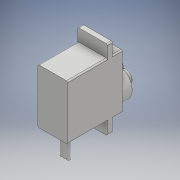
# Autodesk Inventor part: 9g-micro-server
Saved by Autodesk Inventor 2018 (Build 220112000, 112)
## iProperties
Created: 2017-10-10
Part Number: 9g-micro-server
Material: Generic
Document SubType Name: Modeling
Designer: leo2a
Density: 1 g/cm^3
Appearance: Default
Author: leo2a
Autodesk Inventor part; units mm, degrees
ref_plane "YZ Plane" through (0, 0, 0) normal (1, 0, 0) x (0, 1, 0)
ref_plane "XZ Plane" through (0, 0, 0) normal (0, 1, 0) x (-1, 0, 0)
ref_plane "XY Plane" through (0, 0, 0) normal (0, 0, 1) x (1, 0, 0)
sketch "Sketch1" plane through (0, 0, 0) normal (0, 1, 0) x (-1, 0, 0)
  line L0 (-6, 11) -> (-6, -11)
  line L1 (-6, -11) -> (6, -11)
  line L2 (6, -11) -> (6, 11)
  line L3 (6, 11) -> (-6, 11)
  line L4 (-6, 11) -> (6, -11) construction
  line L5 (-6, -11) -> (6, 11) construction
  point P0 (0, 0)
  dimension "d0" = 22
  dimension "d1" = 12
  constraints: 12 end point, 2 midpoint, 2 parallel, 1 perpendicular, 1 vertical
  measures "d0" distance of L0.start L0.end
  measures "d1" distance of L1.end L0.end
extrude "Extrusion1" add sketch "Sketch1" along normal blind 16
sketch "Sketch2" plane through (0, 16, 0) normal (0, 1, 0) x (1, 0, 0)
  line L0 (6, -16) -> (6, 16)
  line L1 (6, 16) -> (-6, 16)
  line L2 (-6, 16) -> (-6, -16)
  line L3 (-6, -16) -> (6, -16)
  line L4 (6, -16) -> (-6, 16) construction
  line L5 (6, 16) -> (-6, -16) construction
  point P0 (0, 0)
  dimension "d4" = 32
  constraints: 12 end point, 2 midpoint, 2 parallel, 1 perpendicular, 1 vertical
  measures "d4" distance of L0.start L0.end
extrude "Extrusion2" add sketch "Sketch2" along normal blind 2
sketch "Sketch3" plane through (0, 18, 0) normal (0, 1, 0) x (1, 0, 0)
  line L0 (6, -11) -> (6, 11)
  line L1 (6, 11) -> (-6, 11)
  line L2 (-6, 11) -> (-6, -11)
  line L3 (-6, -11) -> (6, -11)
  line L4 (6, -11) -> (-6, 11) construction
  line L5 (6, 11) -> (-6, -11) construction
  point P0 (0, 0)
  constraints: 12 end point, 2 midpoint, 2 parallel, 1 perpendicular
extrude "Extrusion3" add sketch "Sketch3" along normal blind 4
sketch "Sketch4" plane through (0, 22, 0) normal (0, 1, 0) x (1, 0, 0)
  line L0 (6, 11) -> (-6, 11) projected
  line L1 (0, 11) -> (0, 5)
  circle A0 centre (0, 5) radius 6
  line L2 (-6, -11) -> (6, -11) projected
  line L3 (0, -11) -> (0, -1)
  circle A1 centre (0, -1) radius 2.5
  point P0 (0, 0)
  dimension "d9" = 6
  dimension "d10" = 10
  dimension "d11" = 5
  constraints: 4 end point, 2 centre point, 2 coincident, 2 midpoint, 2 point on circle, 1 vertical
  measures "d9" distance of L1.start L1.end
  measures "d10" distance of L3.start L3.end
  measures "d11" diameter of A1
extrude "Extrusion4" add sketch "Sketch4" along normal blind 4
sketch "Sketch5" plane through (0, 26, 0) normal (0, 1, 0) x (1, 0, 0)
  circle A0 centre (0, 5) radius 2.5
  point P0 (0, 0)
  dimension "d14" = 5
  constraints: 1 centre point
  measures "d14" diameter of A0
extrude "Extrusion5" add sketch "Sketch5" along normal blind 4
sketch "Sketch6" plane through (0, 30, -5) normal (0, 1, 0) x (1, 0, 0)
  point P0 (0, -5)
  point P1 (0, 0)
hole "Hole1" at (0, 30, -5) direction (0, -1, 0) diameter 1.8 depth 8 tip angle 118 clearance for "Socket Head Cap Screw" size "M1.6" standard "Ansi Metric M Profile"
fillet "Fillet1" radius 0.5 1 edges at (-2.5, 30, -5)
fillet "Fillet2" radius 0.5 9 edges at (6, 20, 11) (6, 8, 11) (-6, 8, 11) (-6, 20, 11) (6, 20, -11) (6, 8, -11) (6, 17, 16) (-6, 17, 16) (6, 17, -16)
fillet "Fillet3" radius 0.5 2 edges at (-6, 20, -11) (-6, 8, -11)
fillet "Fillet4" radius 0.5 2 edges at (2.4451, 24, 0.4792) (-2.4451, 24, 0.4792)
sketch "Sketch7" plane through (5.5, 0, -11) normal (0, 0, -1) x (-1, 0, 0)
  line L0 (5.5, 0) -> (5.5, 5)
  circle A0 centre (5.5, 5) radius 0.635
  line L1 (5.5, 5) -> (4.23, 5)
  circle A1 centre (4.23, 5) radius 0.635
  line L2 (5.5, 5) -> (6.77, 5)
  circle A2 centre (6.77, 5) radius 0.635
  dimension "d28" = 5
  dimension "d29" = 1.27
  dimension "d30" = 1.27
  dimension "d31" = 1.27
  constraints: 6 end point, 3 centre point, 3 coincident, 2 horizontal, 1 vertical
  measures "d28" distance of L0.start L0.end
  measures "d29" diameter of A0
  measures "d30" distance of L1.start L1.end
  measures "d31" distance of L1.start L2.end
extrude "Extrusion6" add sketch "Sketch7" along normal blind 10
body "Solid1"
